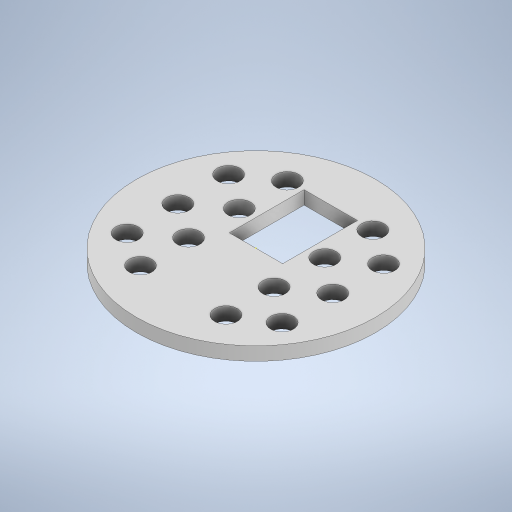
# Autodesk Inventor part: final_탄두낙하산거치대
Saved by Autodesk Inventor 2023 (Build 270158000, 158)
## iProperties
Created: 2023-11-22
Part Number: final_탄두낙하산거치대
Material: 일반
Document SubType Name: Modeling
Designer: rlatk
Density: 1 g/cm^3
Appearance: 기본값
Author: rlatk
Autodesk Inventor part; units mm, degrees
ref_plane "YZ Plane" through (0, 0, 0) normal (1, 0, 0) x (0, 1, 0)
ref_plane "XZ Plane" through (0, 0, 0) normal (0, 1, 0) x (-1, 0, 0)
ref_plane "XY Plane" through (0, 0, 0) normal (0, 0, 1) x (1, 0, 0)
sketch "스케치1" plane through (0, 0, 0) normal (0, 1, 0) x (-1, 0, 0)
  circle A0 centre (0, 0) radius 44.75
  line L0 (0, -44.75) -> (62.1839, -44.75)
  circle A1 centre (16, -27.75) radius 4.25
  circle A2 centre (16, -9.75) radius 4.25
  circle A3 centre (16, 9.25) radius 4.25
  circle A4 centre (16, 27.25) radius 4.25
  circle A5 centre (29, -18.75) radius 4.25
  circle A6 centre (29, 0.25) radius 4.25
  circle A7 centre (29, 19.25) radius 4.25
  line L1 (0, -44.75) -> (0, 44.75)
  circle A8 centre (-16, -27.75) radius 4.25
  circle A9 centre (-16, -9.75) radius 4.25
  circle A10 centre (-16, 9.25) radius 4.25
  circle A11 centre (-16, 27.25) radius 4.25
  circle A12 centre (-29, -18.75) radius 4.25
  circle A13 centre (-29, 0.25) radius 4.25
  circle A14 centre (-29, 19.25) radius 4.25
  dimension "d0" = 89.5
  dimension "d1" = 8.5
  dimension "d2" = 8.5
  dimension "d3" = 8.5
  dimension "d4" = 8.5
  dimension "d5" = 8.5
  dimension "d6" = 8.5
  dimension "d7" = 8.5
  dimension "d8" = 17
  dimension "d9" = 18
  dimension "d10" = 19
  dimension "d11" = 18
  dimension "d12" = 9
  dimension "d13" = 19
  dimension "d14" = 19
  dimension "d15" = 16
  dimension "d16" = 13
  constraints: 15 centre point, 7 symmetric about line, 4 end point, 2 point on circle, 1 coincident, 1 horizontal, 1 perpendicular, 7 other
  measures "d0" diameter of A0
  measures "d1" diameter of A1
  measures "d2" diameter of A2
  measures "d3" diameter of A3
  measures "d4" diameter of A4
  measures "d5" diameter of A5
  measures "d6" diameter of A6
  measures "d7" diameter of A7
  measures "d8" distance from line of A1.centre L0
  measures "d9" distance of A2.centre A1.centre
  measures "d10" distance of A3.centre A2.centre
  measures "d11" distance of A3.centre A4.centre
  measures "d12" vertical distance of A1.centre A5.centre
  measures "d13" distance of A6.centre A5.centre
  measures "d14" distance of A7.centre A6.centre
  measures "d15" distance from line of A1.centre L1
  measures "d16" horizontal distance of A5.centre A1.centre
extrude "돌출1" add sketch "스케치1" along normal blind 5
sketch "스케치2" plane through (0, 5, 0) normal (0, 1, 0) x (1, 0, 0)
  point P0 (0, 0)
sketch "스케치3" plane through (0, 5, 0) normal (0, 1, 0) x (1, 0, 0)
  circle A0 centre (0, 0) radius 44.75 projected
  circle A1 centre (16, 27.75) radius 4.25 projected
  circle A2 centre (16, 9.75) radius 4.25 projected
  circle A3 centre (16, -9.25) radius 4.25 projected
  circle A4 centre (16, -27.25) radius 4.25 projected
  circle A5 centre (29, -19.25) radius 4.25 projected
  circle A6 centre (29, -0.25) radius 4.25 projected
  circle A7 centre (29, 18.75) radius 4.25 projected
  circle A8 centre (-29, -19.25) radius 4.25 projected
  circle A9 centre (-29, -0.25) radius 4.25 projected
  circle A10 centre (-29, 18.75) radius 4.25 projected
  circle A11 centre (-16, -27.25) radius 4.25 projected
  circle A12 centre (-16, -9.25) radius 4.25 projected
  circle A13 centre (-16, 9.75) radius 4.25 projected
  circle A14 centre (-16, 27.75) radius 4.25 projected
  line L0 (10, 0) -> (10, 28)
  line L1 (10, 28) -> (-10, 28)
  line L2 (-10, 28) -> (-10, 0)
  line L3 (0, 0) -> (10, 28) construction
  line L4 (0, 0) -> (-10, 28) construction
  line L5 (10, 0) -> (-10, 0)
  constraints: 12 end point, 2 point on line, 1 midpoint, 1 parallel
extrude "돌출2" cut sketch "스케치3" against normal blind 5 contours L5 L2 L1 L0
